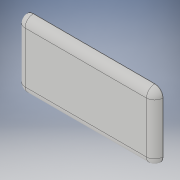
# Autodesk Inventor part: The Cap
Saved by Autodesk Inventor 2019 (Build 230136000, 136)
## iProperties
Created: 2020-02-18
Part Number: The Cap
Material: Generic
Document SubType Name: Modeling
Designer: Delta
Density: 1 g/cm^3
Appearance: Default
Author: Delta
Autodesk Inventor part; units mm, degrees
ref_plane "YZ Plane" through (0, 0, 0) normal (1, 0, 0) x (0, 1, 0)
ref_plane "XZ Plane" through (0, 0, 0) normal (0, 1, 0) x (-1, 0, 0)
ref_plane "XY Plane" through (0, 0, 0) normal (0, 0, 1) x (1, 0, 0)
sketch "Sketch1" plane through (0, 0, 0) normal (0, 0, 1) x (1, 0, 0)
  line L0 (0, 0) -> (102.616, 0)
  line L1 (102.616, 0) -> (102.616, 50.165)
  line L2 (102.616, 50.165) -> (0, 50.165)
  line L3 (0, 50.165) -> (0, 0)
  dimension "d0" = 50.165
  dimension "d1" = 102.616
  constraints: 8 end point, 2 parallel, 1 horizontal, 1 perpendicular
  measures "d0" distance between parallel lines of L2 L0
  measures "d1" distance between parallel lines of L1 L3
extrude "Extrusion1" add sketch "Sketch1" along normal blind 6.35
fillet "Fillet1" radius 6.096 8 edges at (51.308, 0, 6.35) (0, 25.0825, 6.35) (0, 0, 3.175) (102.616, 0, 3.175) (102.616, 25.0825, 6.35) (51.308, 50.165, 6.35) (102.616, 50.165, 3.175) (0, 50.165, 3.175)
body "Solid1"
